# Autodesk Inventor part: LPC1768
Saved by Autodesk Inventor 2015 SP1 (Build 190203100, 203)
## iProperties
Created: 2015-06-25
Part Number: LPC1768
Material: Generic
Document SubType Name: Modeling
Designer: Patrick
Density: 1 g/cm^3
Appearance: LQFP100, LPC1768
Author: Patrick
Autodesk Inventor part; units mm, degrees
ref_plane "YZ Plane" through (0, 0, 0) normal (1, 0, 0) x (0, 1, 0)
ref_plane "XZ Plane" through (0, 0, 0) normal (0, 1, 0) x (-1, 0, 0)
ref_plane "XY Plane" through (0, 0, 0) normal (0, 0, 1) x (1, 0, 0)
sketch "LQFP100, LPC1768_196" plane through (0, 0, 0) normal (0, 0, 1) x (1, 0, 0)
  line L0 (-8.45, -8.45) -> (-8.45, 8.45)
  line L1 (-8.45, 8.45) -> (8.45, 8.45)
  line L2 (8.45, 8.45) -> (8.45, -8.45)
  line L3 (8.45, -8.45) -> (-8.45, -8.45)
  constraints: 8 end point
extrude "Extrusion1" add sketch "LQFP100, LPC1768_196" along normal blind 1
body "Solid1"
